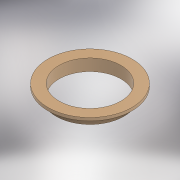
# Autodesk Inventor part: silo_adapter
Saved by Autodesk Inventor 2020 (Build 240168000, 168)
## iProperties
Created: 2020-06-18
Part Number: silo_adapter
Material: Generic
Document SubType Name: Modeling
Designer: pc-konvi
Density: 1 g/cm^3
Appearance: Brindle
Author: pc-konvi
Autodesk Inventor part; units mm, degrees
ref_plane "YZ Plane" through (0, 0, 0) normal (1, 0, 0) x (0, 1, 0)
ref_plane "XZ Plane" through (0, 0, 0) normal (0, 1, 0) x (-1, 0, 0)
ref_plane "XY Plane" through (0, 0, 0) normal (0, 0, 1) x (1, 0, 0)
sketch "Sketch1" plane through (0, 0, 0) normal (0, 0, 1) x (1, 0, 0)
  line L0 (0, 0) -> (23, 0) construction
  line L1 (23, 0) -> (23, 6) construction
  line L2 (23, 6) -> (0, 6) construction
  line L3 (0, 6) -> (0, 0) construction
  line L4 (23, 6) -> (21, 6)
  line L5 (21, 6) -> (21, 0)
  line L6 (21, 0) -> (23, 0)
  line L7 (23, 0) -> (23, 6)
  line L8 (21, 6) -> (28.5, 6)
  line L9 (28.5, 6) -> (28.5, 8)
  line L10 (28.5, 8) -> (21, 8)
  line L11 (21, 8) -> (21, 6)
  dimension "d0" = 23
  dimension "d1" = 6
  dimension "d2" = 2
  dimension "d3" = 7.5
  dimension "d4" = 2
  constraints: 24 end point, 6 parallel, 3 horizontal, 3 perpendicular, 1 point on line
  measures "d0" distance of L2.end L1.end
  measures "d1" distance of L1.end L0.end
  measures "d2" distance of L6.end L5.end
  measures "d3" distance of L10.end L9.end
  measures "d4" distance of L9.end L8.end
revolve "Revolution1" add sketch "Sketch1" angle 360 about axis through (0, 6, 0) along (0, -1, 0)
body "Solid1"
